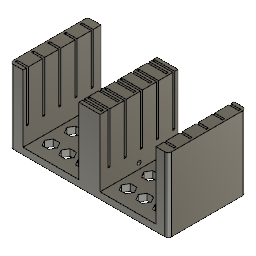
PerfChamberHolder (Autodesk Fusion 360 design; units mm, degrees)
Autodesk Fusion 360 part; units mm, degrees
note: some values were not read from the file. Chosen so that the rebuilt part matches the saved one: which face or edge a step refers to. Set by a fixed rule: which sketch regions a step uses.
sketch "Sketch1" plane through (0, 0, 0) normal (0, 0, 1) x (1, 0, 0)
  line L0 (10, -3) -> (10, -1.2)
  line L1 (10, -1.2) -> (0, -1.2)
  line L2 (0, -1.2) -> (0, -3)
  line L3 (67, -1.2) -> (67, -3)
  line L4 (77, -1.2) -> (67, -1.2)
  line L5 (77, -3) -> (77, -1.2)
  line L6 (67, -3) -> (77, -3)
  line L7 (0, 10.8) -> (0, 9)
  line L8 (10, 10.8) -> (0, 10.8)
  line L9 (10, 9) -> (10, 10.8)
  line L10 (0, 9) -> (10, 9)
  line L11 (67, 10.8) -> (67, 9)
  line L12 (77, 10.8) -> (67, 10.8)
  line L13 (77, 9) -> (77, 10.8)
  line L14 (67, 9) -> (77, 9)
  line L15 (0, 22.8) -> (0, 21)
  line L16 (10, 22.8) -> (0, 22.8)
  line L17 (10, 21) -> (10, 22.8)
  line L18 (0, 21) -> (10, 21)
  line L19 (67, 22.8) -> (67, 21)
  line L20 (77, 22.8) -> (67, 22.8)
  line L21 (77, 21) -> (77, 22.8)
  line L22 (67, 21) -> (77, 21)
  line L23 (0, 40.8) -> (0, 39)
  line L24 (10, 40.8) -> (0, 40.8)
  line L25 (10, 39) -> (10, 40.8)
  line L26 (0, 39) -> (10, 39)
  line L27 (67, 40.8) -> (67, 39)
  line L28 (77, 40.8) -> (67, 40.8)
  line L29 (77, 39) -> (77, 40.8)
  line L30 (67, 39) -> (77, 39)
  line L31 (0, 52.8) -> (0, 51)
  line L32 (10, 52.8) -> (0, 52.8)
  line L33 (10, 51) -> (10, 52.8)
  line L34 (0, 51) -> (10, 51)
  line L35 (67, 52.8) -> (67, 51)
  line L36 (77, 52.8) -> (67, 52.8)
  line L37 (77, 51) -> (77, 52.8)
  line L38 (67, 51) -> (77, 51)
  line L39 (72, 32) -> (72, 33.8)
  line L40 (62, 44) -> (72, 44)
  line L41 (139, 33.8) -> (129, 33.8)
  line L42 (72, 45.8) -> (62, 45.8)
  line L43 (62, 57.8) -> (62, 56)
  line L44 (62, 3.8) -> (62, 2)
  line L45 (72, 14) -> (72, 15.8)
  line L46 (72, 15.8) -> (62, 15.8)
  line L47 (129, 14) -> (139, 14)
  line L48 (62, 56) -> (72, 56)
  line L49 (62, 45.8) -> (62, 44)
  line L50 (139, 45.8) -> (129, 45.8)
  line L51 (139, 2) -> (139, 3.8)
  line L52 (129, 45.8) -> (129, 44)
  line L53 (139, 32) -> (139, 33.8)
  line L54 (129, 15.8) -> (129, 14)
  line L55 (62, 32) -> (72, 32)
  line L56 (139, 3.8) -> (129, 3.8)
  line L57 (129, 2) -> (139, 2)
  line L58 (72, 2) -> (72, 3.8)
  line L59 (139, 57.8) -> (129, 57.8)
  line L60 (139, 15.8) -> (129, 15.8)
  line L61 (72, 56) -> (72, 57.8)
  line L62 (129, 44) -> (139, 44)
  line L63 (129, 32) -> (139, 32)
  line L64 (139, 56) -> (139, 57.8)
  line L65 (129, 3.8) -> (129, 2)
  line L66 (62, 14) -> (72, 14)
  line L67 (62, 2) -> (72, 2)
  line L68 (72, 44) -> (72, 45.8)
  line L69 (62, 33.8) -> (62, 32)
  line L70 (129, 57.8) -> (129, 56)
  line L71 (72, 57.8) -> (62, 57.8)
  line L72 (62, 15.8) -> (62, 14)
  line L73 (72, 3.8) -> (62, 3.8)
  line L74 (139, 44) -> (139, 45.8)
  line L75 (129, 33.8) -> (129, 32)
  line L76 (139, 14) -> (139, 15.8)
  line L77 (129, 56) -> (139, 56)
  line L78 (72, 33.8) -> (62, 33.8)
  line L79 (0, -3) -> (10, -3)
  line L80 (0, 52.8) -> (-2, 52.8)
  line L81 (62, 57.8) -> (62, 60)
  line L82 (62, 60) -> (-2, 60)
  line L83 (-2, 60) -> (10, 60)
  line L84 (10, 60) -> (10, -5)
  line L85 (10, -5) -> (-2, -5)
  line L86 (-2, -5) -> (-2, 60)
  line L87 (62, 60) -> (77, 60)
  line L88 (77, 60) -> (77, -5)
  line L89 (77, -5) -> (62, -5)
  line L90 (62, -5) -> (62, 60)
  line L91 (140, 60) -> (129, 60)
  line L92 (129, 60) -> (129, -5)
  line L93 (129, -5) -> (140, -5)
  line L94 (140, -5) -> (140, 60)
  line L95 (62, 60) -> (60, 60)
  line L96 (60, 60) -> (60, -5)
  line L97 (60, -5) -> (62, -5)
  line L98 (62, -5) -> (62, 60)
  line L99 (77, 60) -> (79, 60)
  line L100 (79, 60) -> (79, -5)
  line L101 (79, -5) -> (77, -5)
  line L102 (77, -5) -> (77, 60)
  line L103 (67, 52.8) -> (60, 52.8)
  line L104 (60, 52.8) -> (60, 51)
  line L105 (60, 51) -> (67, 51)
  line L106 (67, 51) -> (67, 52.8)
  line L107 (67, 40.8) -> (60, 40.8)
  line L108 (60, 40.8) -> (60, 39)
  line L109 (60, 39) -> (67, 39)
  line L110 (67, 39) -> (67, 40.8)
  line L111 (67, 22.8) -> (60, 22.8)
  line L112 (60, 22.8) -> (60, 21)
  line L113 (60, 21) -> (67, 21)
  line L114 (67, 21) -> (67, 22.8)
  line L115 (67, 10.8) -> (60, 10.8)
  line L116 (60, 10.8) -> (60, 9)
  line L117 (60, 9) -> (67, 9)
  line L118 (67, 9) -> (67, 10.8)
  line L119 (67, -1.2) -> (60, -1.2)
  line L120 (60, -1.2) -> (60, -3)
  line L121 (60, -3) -> (67, -3)
  line L122 (67, -3) -> (67, -1.2)
  line L123 (72, 3.8) -> (79, 3.8)
  line L124 (79, 3.8) -> (79, 2)
  line L125 (79, 2) -> (72, 2)
  line L126 (72, 2) -> (72, 3.8)
  line L127 (72, 15.8) -> (79, 15.8)
  line L128 (79, 15.8) -> (79, 14)
  line L129 (79, 14) -> (72, 14)
  line L130 (72, 14) -> (72, 15.8)
  line L131 (72, 33.8) -> (79, 33.8)
  line L132 (79, 33.8) -> (79, 32)
  line L133 (79, 32) -> (72, 32)
  line L134 (72, 32) -> (72, 33.8)
  line L135 (72, 45.8) -> (79, 45.8)
  line L136 (79, 45.8) -> (79, 44)
  line L137 (79, 44) -> (72, 44)
  line L138 (72, 44) -> (72, 45.8)
  line L139 (72, 57.8) -> (79, 57.8)
  line L140 (79, 57.8) -> (79, 56)
  line L141 (79, 56) -> (72, 56)
  line L142 (72, 56) -> (72, 57.8)
  line L143 (-2, 60) -> (10, 60)
  line L144 (10, 60) -> (10, 65)
  line L145 (10, 65) -> (-2, 65)
  line L146 (-2, 65) -> (-2, 60)
  line L147 (60, 60) -> (79, 60)
  line L148 (79, 60) -> (79, 65)
  line L149 (79, 65) -> (60, 65)
  line L150 (60, 65) -> (60, 60)
  line L151 (129, 60) -> (140, 60)
  line L152 (140, 60) -> (140, 65)
  line L153 (140, 65) -> (129, 65)
  line L154 (129, 65) -> (129, 60)
  point P0 (62, 32)
  point P1 (62, 14)
  point P2 (129, 14)
  point P3 (129, 32)
  point P4 (62, 44)
  point P5 (129, 2)
  point P6 (129, 56)
  point P7 (62, 56)
  point P8 (129, 44)
  point P9 (35, -3)
  dimension "d3" = 1.8
  dimension "d8" = 1.8
  dimension "d31" = 2
  dimension "d49" = 65
  dimension "d50" = 65
  dimension "d51" = 5
  constraint horizontal L67
  constraint vertical L58
  constraint horizontal L73
  constraint vertical L44
  constraint perpendicular L0 L79
  constraint perpendicular L31 L80
  constraint perpendicular L71 L81
  constraint perpendicular L81 L82
  constraint horizontal L83
  constraint vertical L84
  constraint horizontal L85
  constraint vertical L86
  constraint horizontal L87
  constraint vertical L88
  constraint horizontal L89
  constraint vertical L90
  constraint horizontal L91
  constraint vertical L92
  constraint horizontal L93
  constraint vertical L94
  constraint horizontal L95
  constraint vertical L96
  constraint horizontal L97
  constraint vertical L98
  constraint horizontal L99
  constraint vertical L100
  constraint horizontal L101
  constraint vertical L102
  constraint horizontal L103
  constraint vertical L104
  constraint horizontal L105
  constraint vertical L106
  constraint coincident L96 L104.end
  constraint horizontal L107
  constraint vertical L108
  constraint horizontal L109
  constraint vertical L110
  constraint coincident L96 L108.end
  constraint horizontal L111
  constraint vertical L112
  constraint horizontal L113
  constraint vertical L114
  constraint coincident L96 L112.end
  constraint horizontal L115
  constraint vertical L116
  constraint horizontal L117
  constraint vertical L118
  constraint coincident L96 L116.end
  constraint horizontal L119
  constraint vertical L120
  constraint horizontal L121
  constraint vertical L122
  constraint horizontal L123
  constraint vertical L124
  constraint horizontal L125
  constraint vertical L126
  constraint coincident L100 L124.end
  constraint horizontal L127
  constraint vertical L128
  constraint horizontal L129
  constraint vertical L130
  constraint coincident L100 L128.end
  constraint horizontal L131
  constraint vertical L132
  constraint horizontal L133
  constraint vertical L134
  constraint coincident L100 L132.end
  constraint horizontal L135
  constraint vertical L136
  constraint horizontal L137
  constraint vertical L138
  constraint coincident L100 L136.end
  constraint horizontal L139
  constraint vertical L140
  constraint horizontal L141
  constraint vertical L142
  constraint coincident L100 L140.end
  constraint horizontal L143
  constraint vertical L144
  constraint horizontal L145
  constraint vertical L146
  constraint horizontal L147
  constraint vertical L148
  constraint horizontal L149
  constraint vertical L150
  constraint horizontal L151
  constraint vertical L152
  constraint horizontal L153
  constraint vertical L154
  measures "d3" distance of L2.end L1.end
  measures "d8" distance of L44.end L44.start
  measures "d31" distance of L87.end L99.end
  measures "d49" distance of L82.end L85.end
  measures "d50" distance of L95.end L96.end
  measures "d51" distance of L95.end L149.end
extrude "Extrude1" add sketch "Sketch1" along normal blind 60 makes body 1 at (140, 16.6667, 20) makes body 2 at (79, 41.6667, 20) makes body 3 at (-2, 41.6667, 20)
sketch "Sketch2" plane through (0, 0, 0) normal (0, 0, -1) x (1, 0, 0)
  line L0 (129, 5) -> (129, -65)
  line L1 (140, -65) -> (140, 5)
  line L2 (140, 5) -> (129, 5)
  line L3 (-2, 5) -> (140, 5)
  line L4 (140, 5) -> (140, -65)
  line L5 (140, -65) -> (-2, -65)
  line L6 (-2, -65) -> (-2, 5)
  line L7 (129, -65) -> (140, -65)
  constraint horizontal L3
  constraint vertical L4
  constraint horizontal L5
  constraint vertical L6
  constraint coincident L1.start L4.end
extrude "Extrude2" add sketch "Sketch2" along normal blind 6 bodies 1 2 3
sketch "Sketch3" plane through (0, 0, 0) normal (0, 0, 1) x (-1, 0, 0)
  line L0 (-79, 5) -> (-129, 5)
  line L1 (-129, 5) -> (-129, -65)
  line L2 (-129, -65) -> (-79, -65)
  line L3 (-22.8868, -45) -> (-25.7735, -50)
  line L4 (-25.7735, -50) -> (-22.8868, -55)
  line L5 (-22.8868, -55) -> (-17.1132, -55)
  line L6 (-17.1132, -55) -> (-14.2265, -50)
  line L7 (-14.2265, -50) -> (-17.1132, -45)
  line L8 (-17.1132, -45) -> (-22.8868, -45)
  line L9 (-29.2265, -50) -> (-32.1132, -45)
  line L10 (-32.1132, -55) -> (-29.2265, -50)
  line L11 (-37.8868, -55) -> (-32.1132, -55)
  line L12 (-32.1132, -45) -> (-37.8868, -45)
  line L13 (-40.7735, -50) -> (-37.8868, -55)
  line L14 (-37.8868, -45) -> (-40.7735, -50)
  line L15 (-44.2265, -50) -> (-47.1132, -45)
  line L16 (-47.1132, -55) -> (-44.2265, -50)
  line L17 (-52.8868, -55) -> (-47.1132, -55)
  line L18 (-47.1132, -45) -> (-52.8868, -45)
  line L19 (-55.7735, -50) -> (-52.8868, -55)
  line L20 (-52.8868, -45) -> (-55.7735, -50)
  line L21 (-14.2265, -30) -> (-17.1132, -25)
  line L22 (-17.1132, -35) -> (-14.2265, -30)
  line L23 (-22.8868, -35) -> (-17.1132, -35)
  line L24 (-17.1132, -25) -> (-22.8868, -25)
  line L25 (-25.7735, -30) -> (-22.8868, -35)
  line L26 (-22.8868, -25) -> (-25.7735, -30)
  line L27 (-29.2265, -30) -> (-32.1132, -25)
  line L28 (-32.1132, -35) -> (-29.2265, -30)
  line L29 (-37.8868, -35) -> (-32.1132, -35)
  line L30 (-32.1132, -25) -> (-37.8868, -25)
  line L31 (-40.7735, -30) -> (-37.8868, -35)
  line L32 (-37.8868, -25) -> (-40.7735, -30)
  line L33 (-44.2265, -30) -> (-47.1132, -25)
  line L34 (-47.1132, -35) -> (-44.2265, -30)
  line L35 (-52.8868, -35) -> (-47.1132, -35)
  line L36 (-47.1132, -25) -> (-52.8868, -25)
  line L37 (-55.7735, -30) -> (-52.8868, -35)
  line L38 (-52.8868, -25) -> (-55.7735, -30)
  line L39 (-14.2265, -10) -> (-17.1132, -5)
  line L40 (-17.1132, -15) -> (-14.2265, -10)
  line L41 (-22.8868, -15) -> (-17.1132, -15)
  line L42 (-17.1132, -5) -> (-22.8868, -5)
  line L43 (-25.7735, -10) -> (-22.8868, -15)
  line L44 (-22.8868, -5) -> (-25.7735, -10)
  line L45 (-29.2265, -10) -> (-32.1132, -5)
  line L46 (-32.1132, -15) -> (-29.2265, -10)
  line L47 (-37.8868, -15) -> (-32.1132, -15)
  line L48 (-32.1132, -5) -> (-37.8868, -5)
  line L49 (-40.7735, -10) -> (-37.8868, -15)
  line L50 (-37.8868, -5) -> (-40.7735, -10)
  line L51 (-44.2265, -10) -> (-47.1132, -5)
  line L52 (-47.1132, -15) -> (-44.2265, -10)
  line L53 (-52.8868, -15) -> (-47.1132, -15)
  line L54 (-47.1132, -5) -> (-52.8868, -5)
  line L55 (-55.7735, -10) -> (-52.8868, -15)
  line L56 (-52.8868, -5) -> (-55.7735, -10)
  line L57 (-10, -20) -> (-129, -20)
  line L58 (-69.5, 8.4492) -> (-69.5, 15)
  line L59 (-98.2265, -50) -> (-101.1133, -55)
  line L60 (-86.1133, -35) -> (-91.8868, -35)
  line L61 (-86.1133, -55) -> (-91.8868, -55)
  line L62 (-91.8868, -35) -> (-94.7735, -30)
  line L63 (-83.2265, -50) -> (-86.1133, -55)
  line L64 (-94.7735, -50) -> (-91.8868, -45)
  line L65 (-83.2265, -30) -> (-86.1133, -35)
  line L66 (-91.8868, -45) -> (-86.1133, -45)
  line L67 (-101.1133, -45) -> (-98.2265, -50)
  line L68 (-106.8868, -35) -> (-109.7735, -30)
  line L69 (-101.1133, -15) -> (-106.8868, -15)
  line L70 (-113.2265, -50) -> (-116.1133, -55)
  line L71 (-116.1133, -45) -> (-113.2265, -50)
  line L72 (-94.7735, -10) -> (-91.8868, -5)
  line L73 (-83.2265, -10) -> (-86.1133, -15)
  line L74 (-91.8868, -25) -> (-86.1133, -25)
  line L75 (-91.8868, -5) -> (-86.1133, -5)
  line L76 (-86.1133, -45) -> (-83.2265, -50)
  line L77 (-91.8868, -55) -> (-94.7735, -50)
  line L78 (-94.7735, -30) -> (-91.8868, -25)
  line L79 (-86.1133, -15) -> (-91.8868, -15)
  line L80 (-86.1133, -5) -> (-83.2265, -10)
  line L81 (-86.1133, -25) -> (-83.2265, -30)
  line L82 (-91.8868, -15) -> (-94.7735, -10)
  line L83 (-124.7735, -50) -> (-121.8868, -45)
  line L84 (-106.8868, -55) -> (-109.7735, -50)
  line L85 (-101.1133, -55) -> (-106.8868, -55)
  line L86 (-106.8868, -25) -> (-101.1133, -25)
  line L87 (-98.2265, -10) -> (-101.1133, -15)
  line L88 (-101.1133, -5) -> (-98.2265, -10)
  line L89 (-121.8868, -35) -> (-124.7735, -30)
  line L90 (-121.8868, -15) -> (-124.7735, -10)
  line L91 (-106.8868, -45) -> (-101.1133, -45)
  line L92 (-106.8868, -5) -> (-101.1133, -5)
  line L93 (-116.1133, -55) -> (-121.8868, -55)
  line L94 (-121.8868, -25) -> (-116.1133, -25)
  line L95 (-116.1133, -35) -> (-121.8868, -35)
  line L96 (-98.2265, -30) -> (-101.1133, -35)
  line L97 (-121.8868, -45) -> (-116.1133, -45)
  line L98 (-101.1133, -35) -> (-106.8868, -35)
  line L99 (-113.2265, -30) -> (-116.1133, -35)
  line L100 (-109.7735, -10) -> (-106.8868, -5)
  line L101 (-116.1133, -15) -> (-121.8868, -15)
  line L102 (-121.8868, -5) -> (-116.1133, -5)
  line L103 (-106.8868, -15) -> (-109.7735, -10)
  line L104 (-121.8868, -55) -> (-124.7735, -50)
  line L105 (-124.7735, -30) -> (-121.8868, -25)
  line L106 (-101.1133, -25) -> (-98.2265, -30)
  line L107 (-116.1133, -5) -> (-113.2265, -10)
  line L108 (-109.7735, -50) -> (-106.8868, -45)
  line L109 (-116.1133, -25) -> (-113.2265, -30)
  line L110 (-124.7735, -10) -> (-121.8868, -5)
  line L111 (-113.2265, -10) -> (-116.1133, -15)
  line L112 (-109.7735, -30) -> (-106.8868, -25)
  line L113 (-79, -65) -> (-79, 5)
  point P0 (-20, -50)
  point P1 (-35, -50)
  point P2 (-50, -50)
  point P3 (-20, -30)
  point P4 (-35, -30)
  point P5 (-50, -30)
  point P6 (-20, -10)
  point P7 (-35, -10)
  point P8 (-50, -10)
  point P9 (-119, -30)
  point P10 (-89, -50)
  point P11 (-89, -30)
  point P12 (-119, -50)
  point P13 (-89, -10)
  point P14 (-104, -50)
  point P15 (-104, -30)
  point P16 (-104, -10)
  point P17 (-119, -10)
  dimension "d16" = -15
  dimension "d17" = 20
  constraint symmetric L3.start L58 L71.start
  constraint symmetric L3.end L58 L70.start
  constraint symmetric L4.end L58 L70.end
  constraint symmetric L5.end L58 L93.end
  constraint symmetric L6.end L58 L83.start
  constraint symmetric L7.end L58 L83.end
  constraint symmetric P0 L58 P12
  constraint symmetric L9.start L58 L84.end
  constraint symmetric L9.end L58 L91.start
  constraint symmetric L10.start L58 L84.start
  constraint symmetric L11.start L58 L59.end
  constraint symmetric L12.end L58 L67.start
  constraint symmetric L13.start L58 L59.start
  constraint symmetric P1 L58 P14
  constraint symmetric L15.start L58 L64.start
  constraint symmetric L15.end L58 L64.end
  constraint symmetric L16.start L58 L61.end
  constraint symmetric L17.start L58 L61.start
  constraint symmetric L18.end L58 L66.end
  constraint symmetric L19.start L58 L63.start
  constraint symmetric P2 L58 P10
  constraint symmetric L21.start L58 L89.end
  constraint symmetric L21.end L58 L94.start
  constraint symmetric L22.start L58 L89.start
  constraint symmetric L23.start L58 L95.start
  constraint symmetric L24.end L58 L94.end
  constraint symmetric L25.start L58 L99.start
  constraint symmetric P3 L58 P9
  constraint symmetric L27.start L58 L68.end
  constraint symmetric L27.end L58 L86.start
  constraint symmetric L28.start L58 L68.start
  constraint symmetric L29.start L58 L96.end
  constraint symmetric L30.end L58 L86.end
  constraint symmetric L31.start L58 L96.start
  constraint symmetric P4 L58 P15
  constraint symmetric L33.start L58 L62.end
  constraint symmetric L33.end L58 L74.start
  constraint symmetric L34.start L58 L60.end
  constraint symmetric L35.start L58 L60.start
  constraint symmetric L36.end L58 L74.end
  constraint symmetric L37.start L58 L65.start
  constraint symmetric P5 L58 P11
  constraint symmetric L39.start L58 L90.end
  constraint symmetric L39.end L58 L102.start
  constraint symmetric L40.start L58 L90.start
  constraint symmetric L41.start L58 L101.start
  constraint symmetric L42.end L58 L102.end
  constraint symmetric L43.start L58 L107.end
  constraint symmetric P6 L58 P17
  constraint symmetric L45.start L58 L100.start
  constraint symmetric L45.end L58 L92.start
  constraint symmetric L46.start L58 L69.end
  constraint symmetric L47.start L58 L69.start
  constraint symmetric L48.end L58 L88.start
  constraint symmetric L49.start L58 L87.start
  constraint symmetric P7 L58 P16
  constraint symmetric L51.start L58 L72.start
  constraint symmetric L51.end L58 L72.end
  constraint symmetric L52.start L58 L79.end
  constraint symmetric L53.start L58 L73.end
  constraint symmetric L54.end L58 L75.end
  constraint symmetric L55.start L58 L73.start
  constraint symmetric P8 L58 P13
extrude "Extrude3" cut sketch "Sketch3" against normal blind 10 contours L3 L4 L5 L6 L7 L8 | L9 L10 L11 L12 L13 L14 | L15 L16 L17 L18 L19 L20 | L21 L22 L23 L24 L25 L26 | L27 L28 L29 L30 L31 L32 | L33 L34 L35 L36 L37 L38 | L39 L40 L41 L42 L43 L44 | L45 L46 L47 L48 L49 L50 | L51 L52 L53 L54 L55 L56 | L59 L67 L84 L85 L91 L108 | L60 L62 L65 L74 L78 L81 | L61 L63 L64 L66 L76 L77 | L68 L86 L96 L98 L106 L112 | L69 L87 L88 L92 L100 L103 | L70 L71 L83 L93 L97 L104 | L72 L73 L75 L79 L80 L82 | L89 L94 L95 L99 L105 L109 | L90 L101 L102 L107 L110 L111 bodies 1
sketch "Sketch4" plane through (0, 0, -6) normal (0, 0, -1) x (1, 0, 0)
  line L0 (86.1133, -15) -> (83.2265, -10)
  line L1 (83.2265, -10) -> (86.1133, -5)
  line L2 (86.1133, -5) -> (91.8868, -5)
  line L3 (91.8868, -5) -> (94.7735, -10)
  line L4 (94.7735, -10) -> (91.8868, -15)
  line L5 (91.8868, -15) -> (86.1133, -15)
  line L6 (116.1133, -55) -> (113.2265, -50)
  line L7 (113.2265, -50) -> (116.1133, -45)
  line L8 (116.1133, -45) -> (121.8868, -45)
  line L9 (121.8868, -45) -> (124.7735, -50)
  line L10 (124.7735, -50) -> (121.8868, -55)
  line L11 (121.8868, -55) -> (116.1133, -55)
  line L12 (55.7735, -30) -> (52.8868, -35)
  line L13 (52.8868, -35) -> (47.1132, -35)
  line L14 (47.1132, -35) -> (44.2265, -30)
  line L15 (44.2265, -30) -> (47.1132, -25)
  line L16 (47.1132, -25) -> (52.8868, -25)
  line L17 (52.8868, -25) -> (55.7735, -30)
  line L18 (25.7735, -30) -> (22.8868, -35)
  line L19 (22.8868, -35) -> (17.1132, -35)
  line L20 (17.1132, -35) -> (14.2265, -30)
  line L21 (14.2265, -30) -> (17.1132, -25)
  line L22 (17.1132, -25) -> (22.8868, -25)
  line L23 (22.8868, -25) -> (25.7735, -30)
  line L24 (22.8868, -45) -> (25.7735, -50)
  line L25 (25.7735, -50) -> (22.8868, -55)
  line L26 (22.8868, -55) -> (17.1132, -55)
  line L27 (17.1132, -55) -> (14.2265, -50)
  line L28 (14.2265, -50) -> (17.1132, -45)
  line L29 (17.1132, -45) -> (22.8868, -45)
  line L30 (40.7735, -30) -> (37.8868, -35)
  line L31 (37.8868, -35) -> (32.1132, -35)
  line L32 (32.1132, -35) -> (29.2265, -30)
  line L33 (29.2265, -30) -> (32.1132, -25)
  line L34 (32.1132, -25) -> (37.8868, -25)
  line L35 (37.8868, -25) -> (40.7735, -30)
  line L36 (55.7735, -10) -> (52.8868, -15)
  line L37 (52.8868, -15) -> (47.1132, -15)
  line L38 (47.1132, -15) -> (44.2265, -10)
  line L39 (44.2265, -10) -> (47.1132, -5)
  line L40 (47.1132, -5) -> (52.8868, -5)
  line L41 (52.8868, -5) -> (55.7735, -10)
  line L42 (121.8868, -25) -> (124.7735, -30)
  line L43 (124.7735, -30) -> (121.8868, -35)
  line L44 (121.8868, -35) -> (116.1133, -35)
  line L45 (116.1133, -35) -> (113.2265, -30)
  line L46 (113.2265, -30) -> (116.1133, -25)
  line L47 (116.1133, -25) -> (121.8868, -25)
  line L48 (101.1133, -15) -> (98.2265, -10)
  line L49 (98.2265, -10) -> (101.1133, -5)
  line L50 (101.1133, -5) -> (106.8868, -5)
  line L51 (106.8868, -5) -> (109.7735, -10)
  line L52 (109.7735, -10) -> (106.8868, -15)
  line L53 (106.8868, -15) -> (101.1133, -15)
  line L54 (91.8868, -25) -> (94.7735, -30)
  line L55 (94.7735, -30) -> (91.8868, -35)
  line L56 (91.8868, -35) -> (86.1133, -35)
  line L57 (86.1133, -35) -> (83.2265, -30)
  line L58 (83.2265, -30) -> (86.1133, -25)
  line L59 (86.1133, -25) -> (91.8868, -25)
  line L60 (106.8868, -55) -> (101.1133, -55)
  line L61 (101.1133, -55) -> (98.2265, -50)
  line L62 (98.2265, -50) -> (101.1133, -45)
  line L63 (101.1133, -45) -> (106.8868, -45)
  line L64 (106.8868, -45) -> (109.7735, -50)
  line L65 (109.7735, -50) -> (106.8868, -55)
  line L66 (40.7735, -10) -> (37.8868, -15)
  line L67 (37.8868, -15) -> (32.1132, -15)
  line L68 (32.1132, -15) -> (29.2265, -10)
  line L69 (29.2265, -10) -> (32.1132, -5)
  line L70 (32.1132, -5) -> (37.8868, -5)
  line L71 (37.8868, -5) -> (40.7735, -10)
  line L72 (55.7735, -50) -> (52.8868, -55)
  line L73 (52.8868, -55) -> (47.1132, -55)
  line L74 (47.1132, -55) -> (44.2265, -50)
  line L75 (44.2265, -50) -> (47.1132, -45)
  line L76 (47.1132, -45) -> (52.8868, -45)
  line L77 (52.8868, -45) -> (55.7735, -50)
  line L78 (40.7735, -50) -> (37.8868, -55)
  line L79 (37.8868, -55) -> (32.1132, -55)
  line L80 (32.1132, -55) -> (29.2265, -50)
  line L81 (29.2265, -50) -> (32.1132, -45)
  line L82 (32.1132, -45) -> (37.8868, -45)
  line L83 (37.8868, -45) -> (40.7735, -50)
  line L84 (25.7735, -10) -> (22.8868, -15)
  line L85 (22.8868, -15) -> (17.1132, -15)
  line L86 (17.1132, -15) -> (14.2265, -10)
  line L87 (14.2265, -10) -> (17.1132, -5)
  line L88 (17.1132, -5) -> (22.8868, -5)
  line L89 (22.8868, -5) -> (25.7735, -10)
  line L90 (86.1133, -55) -> (83.2265, -50)
  line L91 (83.2265, -50) -> (86.1133, -45)
  line L92 (86.1133, -45) -> (91.8868, -45)
  line L93 (91.8868, -45) -> (94.7735, -50)
  line L94 (94.7735, -50) -> (91.8868, -55)
  line L95 (91.8868, -55) -> (86.1133, -55)
  line L96 (106.8868, -35) -> (101.1133, -35)
  line L97 (101.1133, -35) -> (98.2265, -30)
  line L98 (98.2265, -30) -> (101.1133, -25)
  line L99 (101.1133, -25) -> (106.8868, -25)
  line L100 (106.8868, -25) -> (109.7735, -30)
  line L101 (109.7735, -30) -> (106.8868, -35)
  line L102 (116.1133, -5) -> (121.8868, -5)
  line L103 (121.8868, -5) -> (124.7735, -10)
  line L104 (124.7735, -10) -> (121.8868, -15)
  line L105 (121.8868, -15) -> (116.1133, -15)
  line L106 (116.1133, -15) -> (113.2265, -10)
  line L107 (113.2265, -10) -> (116.1133, -5)
  line L108 (-2, -65) -> (140, -65)
  line L109 (140, -65) -> (140, 5)
  line L110 (140, 5) -> (-2, 5)
  line L111 (-2, 5) -> (-2, -65)
  circle A0 centre (69, -30) radius 2.5
  line L112 (69, -30) -> (70.9709, -30)
  line L113 (70.9709, -30) -> (70.9709, -28.462)
  line L114 (70.9709, -30) -> (70.9709, -31.538)
  line L115 (69, -30) -> (74.4999, -30)
  line L116 (75.8999, -32.9) -> (73.0999, -32.9)
  line L117 (73.0999, -32.9) -> (73.0999, -27.1)
  line L118 (73.0999, -27.1) -> (75.8999, -27.1)
  line L119 (75.8999, -27.1) -> (75.8999, -32.9)
  line L120 (75.8999, -32.9) -> (73.0999, -27.1) construction
  line L121 (73.0999, -32.9) -> (75.8999, -27.1) construction
  line L122 (-2, -65) -> (140, 5)
  line L123 (140, -65) -> (-2, 5)
  point P0 (74.4999, -30)
  dimension "d20" = 5
  dimension "d23" = 5.8
  dimension "d24" = 2.8
  constraint coincident A0.centre L112.start
  constraint horizontal L112
  constraint coincident A0 L113.end
  constraint perpendicular L112 L113
  constraint coincident A0 L114.end
  constraint perpendicular L112 L114
  constraint perpendicular L114 L115
  constraint perpendicular L116 L117
  constraint parallel L116 L118
  constraint parallel L117 L119
  constraint horizontal L116
  constraint coincident L120 P0
  constraint coincident L121 P0
  constraint coincident P0 L115.end
  constraint coincident L108.start L111.end
  constraint coincident L109.end L110.start
  constraint coincident L108.end L109.start
  constraint coincident L110.end L111.start
  constraint midpoint A0.centre L122
  measures "d20" diameter of A0
  measures "d23" distance of L116.end L117.end
  measures "d24" distance of L117.end L118.end
extrude "Extrude4" cut sketch "Sketch4" against normal blind 20 contours A0 L114 L122 L123 | L112 L114 L115 L123 | L112 L113 L115 L122 | A0 L122 L123 | A0 L113 L122 L123 bodies 1
extrude "Extrude5" cut sketch "Sketch4" against normal blind 15 contours L116 L117 L118 L119 L122 L123 | L116 L117 L123 | L117 L118 L122 bodies 1
sketch "Sketch6" plane through (79, 0, 0) normal (1, 0, 0) x (0, 1, 0)
  line L0 (15.8, 0) -> (32, 0)
  line L1 (32, 0) -> (32, 70)
  line L2 (32, 70) -> (15.8, 70)
  line L3 (15.8, 70) -> (15.8, 0)
  line L4 (-5, 0) -> (30, 0)
  line L5 (30, 0) -> (30, 5)
  line L6 (30, 5) -> (-5, 5)
  line L7 (-5, 5) -> (-5, 0)
  circle A0 centre (30, 5) radius 1.75
  dimension "d32" = 35
  dimension "d33" = 5
  dimension "d34" = 3.5
  constraint horizontal L4
  constraint vertical L5
  constraint horizontal L6
  constraint vertical L7
  constraint coincident L5.end L6.start
  measures "d32" distance of L4.start L4.end
  measures "d33" distance of L4.start L6.end
  measures "d34" diameter of A0
extrude "Extrude7" cut sketch "Sketch6" against normal blind 8.5 contours L5 L6 A0 | L5 L6 A0 bodies 1
fillet "Fillet1" radius 3 4 edges at (-2, -5, 27) (-2, 65, 27) (140, -5, 27) (140, 65, 27) on bodies 1
sketch "Sketch7" plane through (0, 0, 60) normal (0, 0, 1) x (-1, 0, 0)
  line L0 (-79, -65) -> (-60, -65)
  line L1 (-60, 5) -> (-79, 5)
  line L2 (-79, 5) -> (2, 5)
  line L3 (-38.5, 5) -> (-38.5, 1)
  line L4 (0, 1.9) -> (-77, 1.9)
  line L5 (-77, 1.9) -> (-77, 0.1)
  line L6 (-77, 0.1) -> (0, 0.1)
  line L7 (0, 0.1) -> (0, 1.9)
  line L8 (0, 1.9) -> (-77, 0.1) construction
  line L9 (-77, 1.9) -> (0, 0.1) construction
  line L10 (-79, 5) -> (-79, -65)
  line L11 (-60, -65) -> (-60, 5)
  point P0 (-38.5, 1)
  dimension "d40" = 4
  dimension "d41" = 77
  dimension "d42" = 1.8
  constraint coincident L1.end L2.start
  constraint midpoint L2 L3.start
  constraint perpendicular L2 L3
  constraint horizontal L4
  constraint perpendicular L4 L5
  constraint parallel L4 L6
  constraint parallel L5 L7
  constraint coincident L8 P0
  constraint coincident L9 P0
  constraint coincident P0 L3.end
  measures "d40" distance of L3.start P0
  measures "d41" distance of L5.end L6.end
  measures "d42" distance of L4.end L5.end
extrude "Extrude8" cut sketch "Sketch7" against normal blind 45 contours L4 L6 L7 L11 | L4 L5 L6 L11 bodies 1
pattern_linear "R-Pattern1" count 5 spacing 14.5 along (0, 1, 0) of "Extrude8"
pattern_circular "C-Pattern1" count 2 over 360 about axis through (69, 30, -6) along (0, 0, 1) of "Extrude8"
pattern_linear "R-Pattern2" count 5 spacing 14.5 along (0, -1, 0) of 84 faces at (65.6667, -1.9, 45) (3.3333, -1.9, 45) (65.6667, 12.6, 45) (3.3333, 12.6, 45) (65.6667, 27.1, 45) (3.3333, 27.1, 45) (65.6667, 41.6, 45) (3.3333, 41.6, 45) (65.6667, 56.1, 45) (3.3333, 56.1, 45) (73, 61.9, 45) (135, 61.9, 45) (65.6667, -0.7, 15) (3.3333, -0.7, 15) (65.6667, 13.8, 15) (3.3333, 13.8, 15) (65.6667, 28.3, 15) (3.3333, 28.3, 15) (65.6667, 42.8, 15) (3.3333, 42.8, 15) (65.6667, 57.3, 15) (3.3333, 57.3, 15) (67, 61.3, 15) (132, 61.3, 15) (77, -1.3, 45) (77, 13.2, 45) (77, 27.7, 45) (77, 42.2, 45) (77, 56.7, 45) (61, 61.3, 45) (71.3333, -0.1, 45) (6.6667, -0.1, 45) (71.3333, 14.4, 45) (6.6667, 14.4, 45) (71.3333, 28.9, 45) (6.6667, 28.9, 45) (71.3333, 43.4, 45) (6.6667, 43.4, 45) (71.3333, 57.9, 45) (6.6667, 57.9, 45) (67, 60.1, 45) (132, 60.1, 45) (65.6667, -0.7, 15) (3.3333, -0.7, 15) (65.6667, 13.8, 15) (3.3333, 13.8, 15) (65.6667, 28.3, 15) (3.3333, 28.3, 15) (65.6667, 42.8, 15) (3.3333, 42.8, 15) (65.6667, 57.3, 15) (3.3333, 57.3, 15) (67, 61.3, 15) (132, 61.3, 15) (71.3333, -0.1, 45) (6.6667, -0.1, 45) (71.3333, 14.4, 45) (6.6667, 14.4, 45) (71.3333, 28.9, 45) (6.6667, 28.9, 45) (71.3333, 43.4, 45) (6.6667, 43.4, 45) (71.3333, 57.9, 45) (6.6667, 57.9, 45) (67, 60.1, 45) (132, 60.1, 45) (65.6667, -1.9, 45) (3.3333, -1.9, 45) (65.6667, 12.6, 45) (3.3333, 12.6, 45) (65.6667, 27.1, 45) (3.3333, 27.1, 45) (65.6667, 41.6, 45) (3.3333, 41.6, 45) (65.6667, 56.1, 45) (3.3333, 56.1, 45) (73, 61.9, 45) (135, 61.9, 45) (0, -0.7, 45) (0, 13.8, 45) (0, 28.3, 45) (0, 42.8, 45) (0, 57.3, 45) (138, 60.7, 45) on bodies 1
